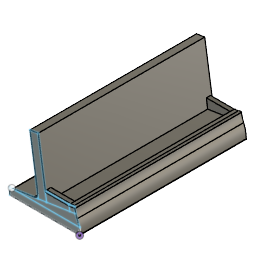
Stand (Autodesk Fusion 360 design; units mm, degrees)
part number: 2026-06-11-17-33-13-659
Autodesk Fusion 360 part; units mm, degrees
sketch "Szkic1" plane through (0, 0, 0) normal (0, 1, 0) x (1, 0, 0)
  line L0 (0, 0) -> (-50, 0) construction
  line L1 (-50, 0) -> (-50, -5) construction
  line L2 (-50, -5) -> (0, -5) construction
  line L3 (0, -5) -> (0, 0) construction
  line L4 (-3, -12) -> (-23.5581, -8.8372) construction
  line L5 (-3, -12) -> (0, -5) construction
  line L6 (-50, -5) -> (0, -5)
  line L7 (0, -5) -> (0, 0)
  line L8 (0, 0) -> (-50, 0)
  line L9 (-50, 0) -> (-50, -5)
  line L10 (-3, -12) -> (0, -5)
  line L11 (-3, -12) -> (-23.5581, -8.8372)
  line L12 (-23.5581, -8.8372) -> (-48.5, -5)
  line L13 (-23.5581, -8.8372) -> (-29.6404, -48.3721)
  line L14 (-3, -12) -> (-3.6082, -15.9535)
  line L15 (-6.9535, -11.3918) -> (-7.5617, -15.3453)
  line L16 (-7.5617, -15.3453) -> (-3.6082, -15.9535)
  line L17 (-29.6404, -48.3721) -> (-35.5706, -47.4597)
  line L18 (-35.5706, -47.4597) -> (-29.4884, -7.9249)
  line L19 (-7.5617, -15.3453) -> (-24.5594, -15.3453)
  dimension "d1" = 20.8
  dimension "d2" = 40
  dimension "d3" = 4
  dimension "d4" = 4
  dimension "d5" = 4
  dimension "d6" = 6
  constraint horizontal L0
  constraint vertical L1
  constraint horizontal L2
  constraint vertical L3
  constraint coincident L0.start L3.end
  constraint horizontal L6
  constraint vertical L7
  constraint horizontal L8
  constraint vertical L9
  constraint parallel L4 L12
  constraint perpendicular L11 L13
  constraint perpendicular L4 L14
  constraint coincident L11 L15.start
  constraint perpendicular L11 L15
  constraint perpendicular L13 L17
  constraint coincident L12 L18.end
  constraint perpendicular L12 L18
  constraint coincident L13 L19.end
  constraint horizontal L19
  measures "d1" distance of L4.start L4.end
  measures "d2" distance of L4.end L13.end
  measures "d3" distance of L4.start L14.end
  measures "d4" distance of L15.start L15.end
  measures "d5" distance of L14 L15
  measures "d6" distance of L13.end L17.end
extrude "Wyciągnięcie proste1" add sketch "Szkic1" along normal blind 4
extrude "Wyciągnięcie proste2" add sketch "Szkic1" along normal blind 115 contours L6 L7 L8 L9 | L6 L10 L11 L12 | L12 L13 L17 L18 | L11 L14 L15 L16
extrude "Wyciągnięcie proste3" add sketch "Szkic1" along normal blind 4 from surface at 115
fillet "Zaokrąglenie1" radius 3 3 edges at (-50, 59.5, 5) (-48.5, 59.5, 5) (-29.4884, 59.5, 7.9249)
fillet "Zaokrąglenie2" radius 1 5 edges at (-16.0605, 0, 15.3453) (-5.585, 0, 15.6494) (-3.6082, 59.5, 15.9535) (-16.0605, 119, 15.3453) (-5.585, 119, 15.6494)
fillet "Zaokrąglenie3" radius 23 2 edges at (-3, 59.5, 12) (0, 59.5, 5)
